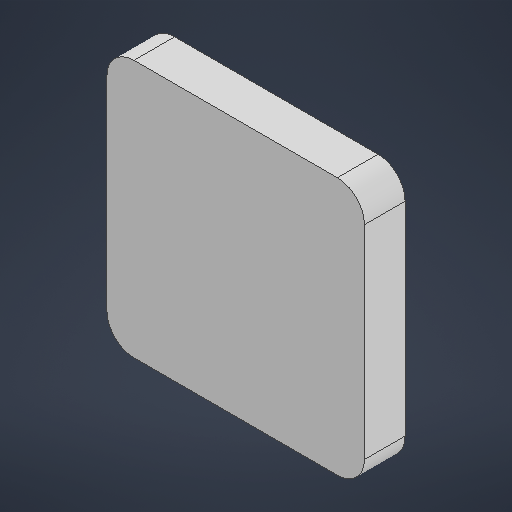
# Autodesk Inventor part: 实体8
Saved by Autodesk Inventor 2025 (Build 290162000, 162)
## iProperties
Created: 2024-12-30
Part Number: 实体8
Material: 常规
Document SubType Name: Modeling
Designer: HZD
Density: 1 g/cm^3
Appearance: 默认
Author: HZD
Autodesk Inventor part; units mm, degrees
ref_plane "YZ Plane" through (0, 0, 0) normal (1, 0, 0) x (0, 1, 0)
ref_plane "XZ Plane" through (0, 0, 0) normal (0, 1, 0) x (-1, 0, 0)
ref_plane "XY Plane" through (0, 0, 0) normal (0, 0, 1) x (1, 0, 0)
sketch "草图1" plane through (0, 0, 0) normal (0, 0, 1) x (1, 0, 0)
  line L0 (9.5, -9.5) -> (-9.5, -9.5)
  line L1 (-9.5, -9.5) -> (-9.5, 9.5)
  line L2 (-9.5, 9.5) -> (9.5, 9.5)
  line L3 (9.5, 9.5) -> (9.5, -9.5)
  line L4 (9.5, -9.5) -> (-9.5, 9.5) construction
  line L5 (-9.5, -9.5) -> (9.5, 9.5) construction
  point P0 (0, 0)
  dimension "d0" = 19
  dimension "d1" = 19
  constraints: 12 end point, 2 midpoint, 2 parallel, 1 horizontal, 1 perpendicular
  measures "d0" distance of L1.end L2.end
  measures "d1" distance of L2.end L0.start
extrude "拉伸1" add sketch "草图1" along normal blind 3
fillet "圆角1" radius 2 4 edges at (-9.5, -9.5, 1.5) (9.5, -9.5, 1.5) (9.5, 9.5, 1.5) (-9.5, 9.5, 1.5)
sketch "草图2" plane through (0, 0, 0) normal (0, 0, -1) x (-1, 0, 0)
  point P0 (0, 0)
